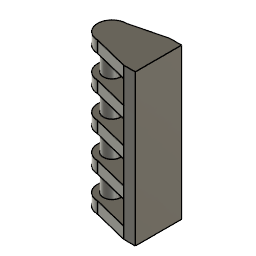
ClipTestRod3mm_v1 (Autodesk Fusion 360 design; units mm, degrees)
Autodesk Fusion 360 part; units mm, degrees
sketch "Sketch1" plane through (0, 0, 0) normal (0, 0, 1) x (1, 0, 0)
  circle A0 centre (0, 0) radius 1.5
  circle A1 centre (0, 0) radius 2.5
  line L0 (0, 0) -> (0, 2.5) construction
  line L1 (0, 0) -> (0, -2.5) construction
  line L2 (0, 0) -> (6, 0) construction
  line L3 (6, -4) -> (6, 4)
  line L4 (6, 4) -> (0, 2.5)
  line L5 (6, -4) -> (0, -2.5)
  line L6 (6, 4) -> (8, 4)
  line L7 (8, 4) -> (8, -4)
  line L8 (8, -4) -> (6, -4)
  line L9 (6, -4) -> (6, 4)
  dimension "d1" = 3
  dimension "d4" = 5
  constraint coincident A0.centre A1.centre
  constraint coincident A1 L0.end
  constraint vertical L0
  constraint coincident A1 L1.end
  constraint parallel L0 L1
  constraint perpendicular L0 L2
  constraint midpoint L2.end L3
  constraint perpendicular L2 L3
  constraint horizontal L6
  constraint vertical L7
  constraint horizontal L8
  constraint vertical L9
  measures "d1" diameter of A0
  measures "d4" diameter of A1
extrude "Extrude1" add sketch "Sketch1" along normal blind 4 contours A0 makes body 1
extrude "Extrude2" add sketch "Sketch1" against normal blind 2 separate body contours A0 | A1 | A1 L3 L4 L5 L9 makes body 2
extrude "Extrude3" add sketch "Sketch1" along normal blind 4 and the other way blind 2 separate body contours L3 L6 L7 L8 L9 makes body 3
combine "Combine1" operation add target body 1 tool bodies 3 2
copy_body "CopyPasteBodies1" bodies 1 makes body 4
move_body "Move1" bodies 4 to x (1, 0, 0) y (0, 1, 0) z (0, 0, 1) at (0, 0, 6)
copy_body "CopyPasteBodies2" bodies 4 1 makes body 5 makes body 6
move_body "Move2" bodies 5 6 to x (1, 0, 0) y (0, 1, 0) z (0, 0, 1) at (0, 0, 12)
extrude "Extrude4" add sketch "Sketch1" along normal blind 2 from surface at 22 contours A0 | A1 | A1 L3 L4 L5 L9 | L3 L6 L7 L8 L9 bodies 5
combine "Combine2" operation add target body 1 tool bodies 6 5 4
